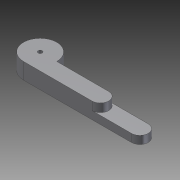
# Autodesk Inventor part: Traba
Saved by Autodesk Inventor 2011 (Build 150239000, 239)
## iProperties
Created: 2014-08-14
Part Number: Traba
Document SubType Name: Modeling
Designer: amatiasq
Density: 1 g/cm^3
Author: amatiasq
Autodesk Inventor part; units mm, degrees
ref_plane "YZ Plane" through (0, 0, 0) normal (1, 0, 0) x (0, 1, 0)
ref_plane "XZ Plane" through (0, 0, 0) normal (0, 1, 0) x (-1, 0, 0)
ref_plane "XY Plane" through (0, 0, 0) normal (0, 0, 1) x (1, 0, 0)
sketch "Boceto1" plane through (0, 0, 0) normal (0, 0, 1) x (1, 0, 0)
  line L0 (0, 0) -> (8, 0)
  line L1 (8, 0) -> (8, 8)
  line L2 (8, 8) -> (0, 8)
  line L3 (0, 8) -> (0, 0)
  line L4 (8, 0) -> (32, 0)
  line L5 (32, 0) -> (32, 4)
  line L6 (32, 4) -> (8, 4)
  line L7 (8, 4) -> (8, 0)
  dimension "d0" = 8
  dimension "d2" = 24
  dimension "d3" = 4
  dimension "d23" = 8
  constraints: 16 end point, 4 parallel, 2 horizontal, 2 perpendicular
  measures "d0" distance of L2.end L1.end
  measures "d2" distance of L6.end L5.end
  measures "d3" distance of L5.end L4.end
  measures "d23" distance of L2.end L0.start
extrude "Extrusión1" add sketch "Boceto1" along normal blind 1.9
fillet "Empalme5" radius 4 3 edges at (0, 0, 0.95) (0, 8, 0.95) (8, 8, 0.95)
fillet "Empalme6" radius 2 2 edges at (32, 4, 0.95) (32, 0, 0.95)
sketch "Boceto2" plane through (0, 0, 1.9) normal (0, 0, 1) x (1, 0, 0)
  arc A0 (8, 4) -> (4, 0) centre (4, 4) ccw projected
  point P0 (0, 0)
  constraints: 1 coincident
hole "Hole1" at (4, 4, 1.9) direction (0, 0, -1) diameter 1 end through all
sketch "Boceto3" plane through (0, 0, 1.9) normal (0, 0, 1) x (1, 0, 0)
  circle A0 centre (4, 4) radius 0.5 projected
  line L0 (8, 4) -> (30, 4) projected
  arc A1 (8, 4) -> (4, 0) centre (4, 4) ccw projected
  line L1 (30, 0) -> (4, 0) projected
  line L2 (22.5, 4) -> (22.5, 0)
  point P0 (0, 0)
  dimension "d19" = 14.5
  constraints: 2 end point, 2 point on line, 1 perpendicular
  measures "d19" distance of L2.start L0.start
extrude "Extrusión2" add sketch "Boceto3" along normal blind 2
fillet "Empalme7" radius 2 2 edges at (22.5, 0, 2.9) (22.5, 4, 2.9)
